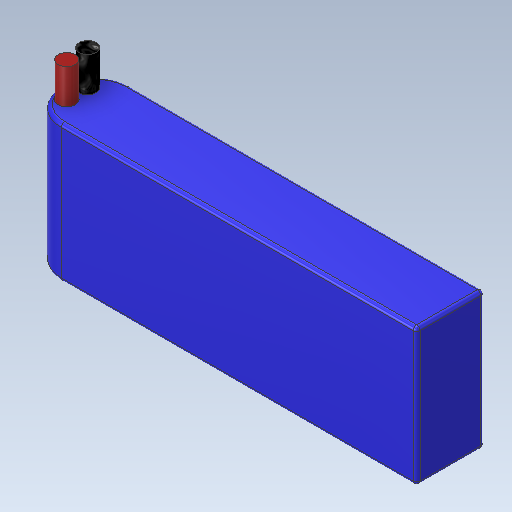
# Autodesk Inventor part: Battery
Saved by Autodesk Inventor 2020 (Build 240168000, 168)
## iProperties
Created: 2019-01-12
Part Number: Battery
Material: Generic
Document SubType Name: Modeling
Designer: LSabe
Density: 1 g/cm^3
Appearance: Default
Author: LSabe
Autodesk Inventor part; units mm, degrees
ref_plane "YZ Plane" through (0, 0, 0) normal (1, 0, 0) x (0, 1, 0)
ref_plane "XZ Plane" through (0, 0, 0) normal (0, 1, 0) x (-1, 0, 0)
ref_plane "XY Plane" through (0, 0, 0) normal (0, 0, 1) x (1, 0, 0)
sketch "Sketch1" plane through (0, 0, 0) normal (0, 1, 0) x (-1, 0, 0)
  line L0 (0, 0) -> (-142.24, 0)
  line L1 (-142.24, 0) -> (-142.24, -24.765)
  line L2 (-142.24, -24.765) -> (0, -24.765)
  line L3 (0, -24.765) -> (0, 0)
  dimension "d0" = 142.24
  dimension "d1" = 24.765
  constraints: 8 end point, 2 parallel, 1 horizontal, 1 perpendicular
  measures "d0" distance of L2.end L1.end
  measures "d1" distance of L1.end L0.end
extrude "Extrusion1" add sketch "Sketch1" along normal blind 50.165
fillet "Fillet1" radius 12.3698 2 edges at (0, 25.0825, 0) (0, 25.0825, -24.765)
fillet "Fillet2" radius 1.27 14 edges at (3.623, 50.165, -3.623) (0, 50.165, -12.3825) (3.623, 50.165, -21.142) (77.3049, 50.165, -24.765) (77.3049, 50.165, 0) (142.24, 50.165, -12.3825) (142.24, 25.0825, 0) (142.24, 25.0825, -24.765) (142.24, 0, -12.3825) (3.623, 0, -21.142) (0, 0, -12.3825) (3.623, 0, -3.623) (77.3049, 0, 0) (77.3049, 0, -24.765)
sketch "Sketch2" plane through (0, 50.165, 0) normal (0, 1, 0) x (1, 0, 0)
  line L0 (12.3698, 23.495) -> (140.97, 23.495) projected
  arc A0 (12.3698, 23.495) -> (1.27, 12.3952) centre (12.3698, 12.3952) ccw projected
  line L1 (1.27, 12.3698) -> (1.27, 12.3952) projected
  arc A1 (1.27, 12.3698) -> (12.3698, 1.27) centre (12.3698, 12.3698) ccw projected
  line L2 (140.97, 1.27) -> (12.3698, 1.27) projected
  line L3 (140.97, 23.495) -> (140.97, 1.27) projected
  line L4 (12.3698, 12.3698) -> (5.7707, 16.1798)
  line L5 (12.3698, 12.3698) -> (19.9898, 12.3698) construction
  line L6 (12.3698, 12.3698) -> (5.7707, 8.5598)
  line L7 (12.3698, 12.3698) -> (19.9898, 12.3698) construction
  circle A2 centre (5.7707, 8.5598) radius 3.175
  circle A3 centre (5.7707, 16.1798) radius 3.175
  point P0 (0, 0)
  dimension "d6" = 7.62
  dimension "d7" = 150
  dimension "d8" = 7.62
  dimension "d9" = 150
  dimension "d10" = 6.35
  dimension "d11" = 6.35
  constraints: 8 end point, 2 centre point, 2 coincident, 2 equal length, 2 horizontal
  measures "d6" distance of L4.start L4.end
  measures "d7" angle of L5 L4
  measures "d8" distance of L4.start L6.end
  measures "d9" angle of L6 L7
  measures "d10" diameter of A2
  measures "d11" diameter of A3
extrude "Extrusion2" add sketch "Sketch2" along normal blind 12.7 contours A3 | A2
body "Solid1"
